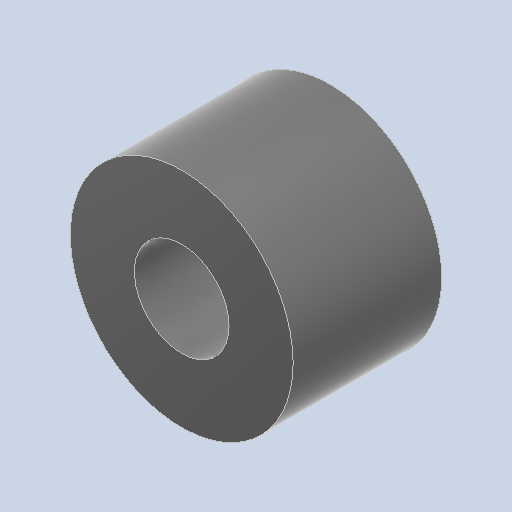
# Autodesk Inventor part: SPACER,ROCKER,ELEVATOR
Saved by Autodesk Inventor 2025.2 (Build 292293000, 293)
## iProperties
ILogicPurgeVersion: 0.0.0.0
Created: 2025-02-01
Part Number: SPACER,ROCKER,ELEVATOR
Material: Nylon 6/6
Document SubType Name: Modeling
Designer: Johna
Density: 1.13 g/cm^3
Appearance: Smooth - Black
ModelCat: Uncategorized
Author: Johna
Autodesk Inventor part; units mm, degrees
ref_plane "YZ Plane" through (0, 0, 0) normal (1, 0, 0) x (0, 1, 0)
ref_plane "XZ Plane" through (0, 0, 0) normal (0, 1, 0) x (-1, 0, 0)
ref_plane "XY Plane" through (0, 0, 0) normal (0, 0, 1) x (1, 0, 0)
sketch "Sketch1" plane through (0, 0, 0) normal (0, 0, 1) x (1, 0, 0)
  circle A0 centre (0, 0) radius 4.045
  circle A1 centre (0, 0) radius 9.525
  dimension "d0" = 8.0899
  dimension "d1" = 19.05
  constraints: 2 centre point, 2 coincident
  measures "d0" diameter of A0
  measures "d1" diameter of A1
extrude "Extrusion1" add sketch "Sketch1" along normal blind 12.7
body "Solid1"
